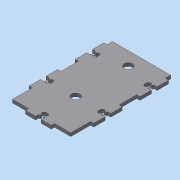
# Autodesk Inventor part: Y-Shafts-Holder_Front-Outer
Saved by Autodesk Inventor 2016 SP1 (Build 200210100, 210)
## iProperties
Created: 2016-01-21
Part Number: Y-Shafts-Holder_Front-Outer
Material: Generic
Document SubType Name: Modeling
Designer: Mohamed A.
Density: 1 g/cm^3
Appearance: Default
Author: Mohamed A.
Autodesk Inventor part; units mm, degrees
ref_plane "YZ Plane" through (0, 0, 0) normal (1, 0, 0) x (0, 1, 0)
ref_plane "XZ Plane" through (0, 0, 0) normal (0, 1, 0) x (-1, 0, 0)
ref_plane "XY Plane" through (0, 0, 0) normal (0, 0, 1) x (1, 0, 0)
sketch "Sketch1" plane through (0, 0, 0) normal (0, 0, 1) x (1, 0, 0)
  line L0 (-22.8574, 44.4294) -> (22.8574, 44.4294)
  line L1 (10.3429, -56) -> (10.3429, -59)
  line L2 (2.65, -59) -> (2.65, -56)
  line L3 (2.65, -56) -> (1.5, -56)
  line L4 (1.5, -56) -> (1.5, -54)
  line L5 (1.5, -54) -> (2.65, -54)
  line L6 (2.65, -54) -> (2.65, -51.6)
  line L7 (2.65, -51.6) -> (1.5, -51.6)
  line L8 (1.5, -51.6) -> (1.5, -51)
  line L9 (1.5, -51) -> (-1.5, -51)
  line L10 (-1.5, -51) -> (-1.5, -51.6)
  line L11 (-1.5, -51.6) -> (-2.65, -51.6)
  line L12 (-2.65, -51.6) -> (-2.65, -54)
  line L13 (-2.65, -54) -> (-1.5, -54)
  line L14 (-1.5, -56) -> (-2.65, -56)
  line L15 (-1.5, -54) -> (-1.5, -56)
  line L16 (-2.65, -56) -> (-2.65, -59)
  line L17 (-10.3429, -56) -> (-10.3429, -59)
  line L18 (0, -51.179) -> (0, -65.7621) construction
  line L19 (10.3429, -59) -> (2.65, -59)
  line L20 (-2.65, -59) -> (-10.3429, -59)
  line L21 (-24.2882, 0) -> (26.7754, 0) construction
  circle A0 centre (0, -24.4294) radius 3.9
  circle A1 centre (0, 24.4294) radius 3.9
  line L22 (22.8574, -56) -> (22.8574, -34.4294)
  line L23 (22.8574, -34.4294) -> (25.8574, -34.4294)
  line L24 (25.8574, -27.0794) -> (22.8574, -27.0794)
  line L25 (22.8574, -27.0794) -> (22.8574, -25.9294)
  line L26 (22.8574, -25.9294) -> (20.8574, -25.9294)
  line L27 (20.8574, -25.9294) -> (20.8574, -27.0794)
  line L28 (20.8574, -27.0794) -> (18.4574, -27.0794)
  line L29 (18.4574, -27.0794) -> (18.4574, -25.9294)
  line L30 (18.4574, -25.9294) -> (17.8574, -25.9294)
  line L31 (17.8574, -25.9294) -> (17.8574, -22.9294)
  line L32 (17.8574, -22.9294) -> (18.4574, -22.9294)
  line L33 (18.4574, -22.9294) -> (18.4574, -21.7794)
  line L34 (18.4574, -21.7794) -> (20.8574, -21.7794)
  line L35 (20.8574, -21.7794) -> (20.8574, -22.9294)
  line L36 (20.8574, -22.9294) -> (22.8574, -22.9294)
  line L37 (22.8574, -22.9294) -> (22.8574, -21.7794)
  line L38 (22.8574, -21.7794) -> (25.8574, -21.7794)
  line L39 (22.8574, -56) -> (10.3429, -56)
  line L40 (39.0531, -24.4294) -> (-31.8887, -24.4294) construction
  line L41 (25.8574, -14.4294) -> (22.8574, -14.4294)
  line L42 (25.8574, -27.0794) -> (25.8574, -34.4294)
  line L43 (25.8574, -14.4294) -> (25.8574, -21.7794)
  line L44 (22.8574, 44.4294) -> (22.8574, 34.4294)
  line L45 (22.8574, 34.4294) -> (25.8574, 34.4294)
  line L46 (25.8574, 27.0794) -> (22.8574, 27.0794)
  line L47 (22.8574, 27.0794) -> (22.8574, 25.9294)
  line L48 (22.8574, 25.9294) -> (20.8574, 25.9294)
  line L49 (20.8574, 25.9294) -> (20.8574, 27.0794)
  line L50 (20.8574, 27.0794) -> (18.4574, 27.0794)
  line L51 (18.4574, 27.0794) -> (18.4574, 25.9294)
  line L52 (18.4574, 25.9294) -> (17.8574, 25.9294)
  line L53 (17.8574, 25.9294) -> (17.8574, 22.9294)
  line L54 (17.8574, 22.9294) -> (18.4574, 22.9294)
  line L55 (18.4574, 22.9294) -> (18.4574, 21.7794)
  line L56 (18.4574, 21.7794) -> (20.8574, 21.7794)
  line L57 (20.8574, 21.7794) -> (20.8574, 22.9294)
  line L58 (20.8574, 22.9294) -> (22.8574, 22.9294)
  line L59 (22.8574, 22.9294) -> (22.8574, 21.7794)
  line L60 (22.8574, 21.7794) -> (25.8574, 21.7794)
  line L61 (25.8574, 14.4294) -> (22.8574, 14.4294)
  line L62 (25.8574, 27.0794) -> (25.8574, 34.4294)
  line L63 (25.8574, 14.4294) -> (25.8574, 21.7794)
  line L64 (22.8574, 14.4294) -> (22.8574, -14.4294)
  line L65 (0, 77.8205) -> (0, -95.1737) construction
  line L66 (-22.8574, -56) -> (-22.8574, -34.4294)
  line L67 (-22.8574, -34.4294) -> (-25.8574, -34.4294)
  line L68 (-25.8574, -27.0794) -> (-22.8574, -27.0794)
  line L69 (-22.8574, -27.0794) -> (-22.8574, -25.9294)
  line L70 (-22.8574, -25.9294) -> (-20.8574, -25.9294)
  line L71 (-20.8574, -25.9294) -> (-20.8574, -27.0794)
  line L72 (-20.8574, -27.0794) -> (-18.4574, -27.0794)
  line L73 (-18.4574, -27.0794) -> (-18.4574, -25.9294)
  line L74 (-18.4574, -25.9294) -> (-17.8574, -25.9294)
  line L75 (-17.8574, -25.9294) -> (-17.8574, -22.9294)
  line L76 (-17.8574, -22.9294) -> (-18.4574, -22.9294)
  line L77 (-18.4574, -22.9294) -> (-18.4574, -21.7794)
  line L78 (-18.4574, -21.7794) -> (-20.8574, -21.7794)
  line L79 (-20.8574, -21.7794) -> (-20.8574, -22.9294)
  line L80 (-20.8574, -22.9294) -> (-22.8574, -22.9294)
  line L81 (-22.8574, -22.9294) -> (-22.8574, -21.7794)
  line L82 (-22.8574, -21.7794) -> (-25.8574, -21.7794)
  line L83 (-25.8574, -14.4294) -> (-22.8574, -14.4294)
  line L84 (-25.8574, -27.0794) -> (-25.8574, -34.4294)
  line L85 (-25.8574, -14.4294) -> (-25.8574, -21.7794)
  line L86 (-25.8574, 14.4294) -> (-22.8574, 14.4294)
  line L87 (-25.8574, 14.4294) -> (-25.8574, 21.7794)
  line L88 (-22.8574, 21.7794) -> (-25.8574, 21.7794)
  line L89 (-22.8574, 22.9294) -> (-22.8574, 21.7794)
  line L90 (-20.8574, 22.9294) -> (-22.8574, 22.9294)
  line L91 (-20.8574, 21.7794) -> (-20.8574, 22.9294)
  line L92 (-18.4574, 21.7794) -> (-20.8574, 21.7794)
  line L93 (-18.4574, 22.9294) -> (-18.4574, 21.7794)
  line L94 (-17.8574, 22.9294) -> (-18.4574, 22.9294)
  line L95 (-17.8574, 25.9294) -> (-17.8574, 22.9294)
  line L96 (-18.4574, 25.9294) -> (-17.8574, 25.9294)
  line L97 (-18.4574, 27.0794) -> (-18.4574, 25.9294)
  line L98 (-20.8574, 27.0794) -> (-18.4574, 27.0794)
  line L99 (-20.8574, 25.9294) -> (-20.8574, 27.0794)
  line L100 (-22.8574, 25.9294) -> (-20.8574, 25.9294)
  line L101 (-22.8574, 27.0794) -> (-22.8574, 25.9294)
  line L102 (-25.8574, 27.0794) -> (-22.8574, 27.0794)
  line L103 (-25.8574, 27.0794) -> (-25.8574, 34.4294)
  line L104 (-22.8574, 34.4294) -> (-25.8574, 34.4294)
  line L105 (-22.8574, 44.4294) -> (-22.8574, 34.4294)
  line L106 (-22.8574, 14.4294) -> (-22.8574, -14.4294)
  line L107 (-22.8574, -56) -> (-10.3429, -56)
  line L108 (-37.0496, 24.4294) -> (41.724, 24.4294) construction
  point P0 (0, 0)
  dimension "d4" = 3
  dimension "d6" = 3
  dimension "d7" = 2.4
  dimension "d10" = 5.3
  dimension "d11" = 8
  dimension "d12" = 5
  dimension "d13" = 20.6859
  dimension "d14" = 7.8
  dimension "d15" = 34.5706
  dimension "d16" = 7.8
  dimension "d24" = 3
  dimension "d26" = 51.7147
  dimension "d29" = 48.8588
  dimension "d31" = 3
  dimension "d32" = 8
  dimension "d33" = 5.3
  dimension "d36" = 20
  dimension "d37" = 20
  dimension "d38" = 10
  dimension "d39" = 103.4294
  constraints: 218 end point, 72 point on line, 42 symmetric about line, 27 perpendicular, 9 collinear, 9 equal length, 8 horizontal, 7 vertical, 2 centre point, 2 parallel, 15 other
  measures "d4" distance of L1.end L1.start
  measures "d6" distance of L8.end L9.end
  measures "d7" distance of L5.end L6.end
  measures "d10" distance between parallel lines of L12 L6
  measures "d11" distance between parallel lines of L19 L9
  measures "d12" distance between parallel lines of L19 L5
  measures "d13" distance between parallel lines of L17 L1
  measures "d14" diameter of A0
  measures "d15" distance from line of L19 A0.centre
  measures "d16" diameter of A1
  measures "d24" distance between parallel lines of L20 L107
  measures "d26" distance between parallel lines of L42 L84
  measures "d29" distance of A0.centre A1.centre
  measures "d31" distance of L95.start L94.start
  measures "d32" distance between parallel lines of L87 L95
  measures "d33" distance between parallel lines of L92 L98
  measures "d36" distance between parallel lines of L23 L41
  measures "d37" distance between parallel lines of L61 L45
  measures "d38" distance between parallel lines of L104 L0
  measures "d39" distance between parallel lines of L20 L0
extrude "Extrusion1" add sketch "Sketch1" along normal blind 3
equation "\"d13\" = 0.4 * d26"
body "Solid1"
